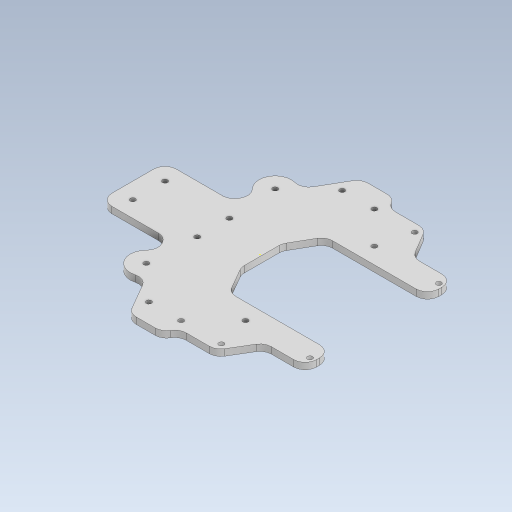
# Autodesk Inventor part: Fix Konektor Casis
Saved by Autodesk Inventor 2023.5 (Build 275446000, 446)
## iProperties
Created: 2025-10-01
Part Number: Fix Konektor Casis
Material: Generic
Document SubType Name: Modeling
Designer: Guntur
Density: 1 g/cm^3
Appearance: Default
Author: Guntur
## iProperties of the stored document Fix Konektor Casis_3DPrint.ipt
Created: 2025-10-18
Part Number: Fix Konektor Casis_3DPrint
Material: Generic
Document SubType Name: Modeling
Designer: Guntur
Density: 1 g/cm^3
Appearance: Default
Author: Guntur
Autodesk Inventor part; units mm, degrees
ref_plane "YZ Plane" through (0, 0, 0) normal (1, 0, 0) x (0, 1, 0)
ref_plane "XZ Plane" through (0, 0, 0) normal (0, 1, 0) x (-1, 0, 0)
ref_plane "XY Plane" through (0, 0, 0) normal (0, 0, 1) x (1, 0, 0)
sketch "Sketch1" plane through (0, 0, 0) normal (0, 1, 0) x (-1, 0, 0)
  line L0 (121, 0) -> (-97, 0) construction
  circle A0 centre (29, -10) radius 1.6
  circle A1 centre (69, -10) radius 1.6
  circle A2 centre (9, -60) radius 1.6
  circle A3 centre (-11, -60) radius 1.6
  line L1 (79, 0) -> (79, -20)
  line L2 (79, -20) -> (39, -20)
  line L3 (9, -71.9615) -> (-11, -71.9615)
  circle A4 centre (-31, -40) radius 1.6
  line L4 (-11, -71.9615) -> (-15.0192, -65)
  line L5 (-11, -71.9615) -> (19, -71.9615) construction
  circle A5 centre (-71, -40) radius 1.6
  line L6 (-49, -45.9808) -> (-81, -45.9808)
  line L7 (-81, -45.9808) -> (-81, -29.9998)
  line L8 (-81, -29.9998) -> (-11, -29.9998)
  line L9 (-11, -29.9998) -> (-1, -12.6793)
  line L10 (-1, -12.6793) -> (-1, 0)
  circle A6 centre (29, 10) radius 1.6
  circle A7 centre (69, 10) radius 1.6
  circle A8 centre (9, 60) radius 1.6
  circle A9 centre (-11, 60) radius 1.6
  line L11 (79, 0) -> (79, 20)
  line L12 (79, 20) -> (39, 20)
  line L13 (9, 71.9615) -> (-11, 71.9615)
  circle A10 centre (-31, 40) radius 1.6
  line L14 (-11, 71.9615) -> (-15.0192, 65)
  line L15 (-11, 71.9615) -> (19, 71.9615) construction
  circle A11 centre (-71, 40) radius 1.6
  line L16 (-49, 45.9808) -> (-81, 45.9808)
  line L17 (-81, 45.9808) -> (-81, 29.9998)
  line L18 (-81, 29.9998) -> (-11, 29.9998)
  line L19 (-11, 29.9998) -> (-1, 12.6793)
  line L20 (-1, 12.6793) -> (-1, 0)
  line L21 (-81, -45.9808) -> (-74, -45.9808)
  line L22 (-74, -45.9808) -> (-74, -29.9998)
  line L23 (-74, 29.9998) -> (-74, 45.9808)
  circle A12 centre (30.6, 40) radius 1.6
  arc A13 (33.0505, 30.3049) -> (23.429, 46.9697) centre (30.6, 40) ccw
  circle A14 centre (30.6, -40) radius 1.6
  arc A15 (23.429, -46.9697) -> (33.0505, -30.3049) centre (30.6, -40) ccw
  line L24 (39, 20) -> (33.0505, 30.3049)
  line L25 (23.429, 46.9697) -> (9, 71.9615)
  line L26 (39, -20) -> (33.0505, -30.3049)
  line L27 (23.429, -46.9697) -> (9, -71.9615)
  circle A16 centre (-36, 60) radius 1.6
  line L28 (-11, 60) -> (-11, 61.6)
  line L29 (-15.0192, 65) -> (-37.6, 65)
  line L30 (-37.6, 65) -> (-49, 45.9808)
  circle A17 centre (-36, -60) radius 1.6
  line L31 (-15.0192, -65) -> (-37.6, -65)
  line L32 (-37.6, -65) -> (-49, -45.9808)
  point P0 (0, 0)
  point P1 (-26, -45.9808)
  point P2 (-26, 45.9808)
  dimension "d0" = 3.2
  dimension "d3" = 3.2
  dimension "d5" = 3.2
  dimension "d6" = 50
  dimension "d15" = 20
  dimension "d16" = 40
  dimension "d18" = 20
  dimension "d25" = 3.2
  dimension "d27" = 40
  dimension "d28" = 120
  dimension "d29" = 3.2
  dimension "d30" = 40
  dimension "d31" = 55
  dimension "d32" = 15.981
  dimension "d33" = 120
  dimension "d36" = 3.2
  dimension "d37" = 30
  dimension "d38" = 20
  dimension "d39" = 3.2
  dimension "d40" = 25
  constraints: 66 end point, 22 symmetric about line, 17 centre point, 8 point on line, 6 horizontal, 4 perpendicular, 4 point on circle, 2 coincident, 2 vertical, 1 parallel, 1 vertical alignment, 11 other
  measures "d0" diameter of A0
  measures "d3" diameter of A1
  measures "d5" diameter of A2
  measures "d6" vertical distance of A2.centre A0.centre
  measures "d15" distance of L1.start L1.end
  measures "d16" distance of L1.end L2.end
  measures "d18" distance of L3.start L3.end
  measures "d25" diameter of A4
  measures "d27" distance from line of L0 A4.centre
  measures "d28" angle of L5 L4
  measures "d29" diameter of A5
  measures "d30" distance of A5.centre A4.centre
  measures "d31" distance of point (-26, -45.981) L6.end
  measures "d32" distance of L6.end L7.end
  measures "d33" angle of L9 L8
  measures "d36" diameter of A12
  measures "d37" vertical distance of A12.centre A6.centre
  measures "d38" diameter of A13
  measures "d39" diameter of A16
  measures "d40" distance of A16.centre L28.start
extrude "Extrusion1" add sketch "Sketch1" along normal blind 4
sketch "Sketch2" plane through (0, 4, 0) normal (0, 1, 0) x (1, 0, 0)
  point P0 (0, 0)
extrude "Extrusion2" cut sketch "Sketch1" along normal blind 4 contours L6 L7 L8 L22 | L23 L18 L17 L16
fillet "Fillet1" radius 7 26 edges at (49, 2, 45.9808) (37.6, 2, 65) (74, 2, 45.9808) (74, 2, 29.9998) (1, 2, 12.6793) (1, 2, -12.6793) (11, 2, -29.9998) (11, 2, 29.9998) (74, 2, -29.9998) (49, 2, -45.9808) (74, 2, -45.9808) (37.6, 2, -65) (15.0192, 2, -65) (11, 2, -71.9615) (-9, 2, -71.9615) (-23.429, 2, -46.9697) (-33.0505, 2, -30.3049) (-39, 2, -20) (-79, 2, -20) (-79, 2, 20) (-33.0505, 2, 30.3049) (-39, 2, 20) (-23.429, 2, 46.9697) (-9, 2, 71.9615) (11, 2, 71.9615) (15.0192, 2, 65)
body "Solid1"
